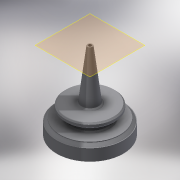
# Autodesk Inventor part: nozzle-tip1-0402
Saved by Autodesk Inventor 2016 (Build 200138000, 138)
## iProperties
Created: 2015-05-09
Part Number: nozzle-tip1-0402
Material: Steel, Mild
Document SubType Name: Modeling
Designer: ax
Density: 7.85 g/cm^3
Appearance: Semi-Polished
Mass: 6.33937 g
Surface Area: 8.38326 cm^2
Volume: 0.807563 cm^3
Author: ax
Autodesk Inventor part; units mm, degrees
ref_plane "YZ Plane" through (0, 0, 0) normal (1, 0, 0) x (0, 1, 0)
ref_plane "XZ Plane" through (0, 0, 0) normal (0, 1, 0) x (-1, 0, 0)
ref_plane "XY Plane" through (0, 0, 0) normal (0, 0, 1) x (1, 0, 0)
sketch "Sketch1" plane through (0, 0, 0) normal (0, 0, 1) x (1, 0, 0)
  point P0 (0, 0)
sketch "Sketch2" plane through (0, 0, 0) normal (0, 0, 1) x (1, 0, 0)
  circle A0 centre (0, 0) radius 6.975
  circle A1 centre (0, 0) radius 2.5
  dimension "d0" = 13.95
  dimension "d1" = 5
  constraints: 2 centre point, 2 coincident
  measures "d0" diameter of A0
  measures "d1" diameter of A1
extrude "Extrusion1" add sketch "Sketch2" along normal blind 2
sketch "Sketch3" plane through (0, 0, 2) normal (0, 0, 1) x (1, 0, 0)
  circle A0 centre (0, 0) radius 6
  dimension "d9" = 12
  constraints: 1 centre point, 1 coincident
  measures "d9" diameter of A0
extrude "Extrusion2" add sketch "Sketch3" along normal blind 1
sketch "Sketch4" plane through (0, 0, 3) normal (0, 0, 1) x (1, 0, 0)
  circle A0 centre (0, 0) radius 4
  dimension "nozzleInner" = 8
  constraints: 1 centre point, 1 coincident
  measures "nozzleInner" diameter of A0
extrude "Extrusion3" add sketch "Sketch4" along normal blind 2.25
chamfer "Chamfer1" distance 0.8 angle 45 1 edges at (-6, 0, 2)
sketch "Sketch5" plane through (0, 0, 5.25) normal (0, 0, 1) x (1, 0, 0)
  circle A0 centre (0, 0) radius 6
  dimension "d24" = 12
  constraints: 1 centre point, 1 coincident
  measures "d24" diameter of A0
extrude "Extrusion4" add sketch "Sketch5" along normal blind 1.5
ref_plane "Work Plane2" through (0, 0, 21.75) normal (0, 0, 1) x (1, 0, 0)
sketch "Sketch8" plane through (0, 0, 21.75) normal (0, 0, 1) x (1, 0, 0)
  circle A0 centre (0, 0) radius 0.5
  circle A1 centre (0, 0) radius 0.75
  dimension "d39" = 1
  dimension "d40" = 1.5
  constraints: 2 centre point, 2 coincident
  measures "d39" diameter of A0
  measures "d40" diameter of A1
extrude "Extrusion7" add sketch "Sketch8" against normal blind 15
draft "FaceDraft1" angle 7 pull direction (0, 0, 1) faces at (0.7476, -0.0603, 11.75) fixed edges at (-0.75, 0, 21.75)
chamfer "Chamfer2" distance 0.4 angle 45 5 edges at (-6, 0, 5.25) (-6, 0, 6.75) (-4, 0, 3) (-4, 0, 5.25) (-2.5918, 0, 6.75)
equation "\"d1\" = di"
equation "\"d4\" = d10"
equation "\"nozzleInner\" = 0.5 * dO"
equation "\"d39\" = iTip"
equation "\"d40\" = oTip"
equation "\"iTip\" = 1"
equation "\"oTip\" = 1.5"
equation "\"di\" = 5"
equation "\"d10\" = 2"
equation "\"dO\" = 16"
body "Solid1"
